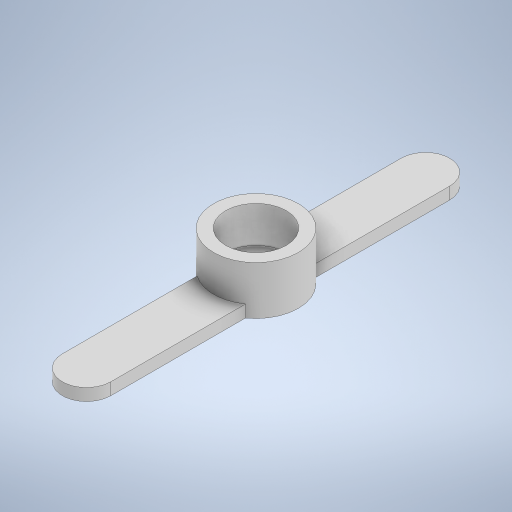
# Autodesk Inventor part: ServoWings
Saved by Autodesk Inventor 2024.2 (Build 282272000, 272)
## iProperties
Created: 2024-05-04
Part Number: ServoWings
Material: Generic
Document SubType Name: Modeling
Designer: ringl
Density: 1 g/cm^3
Appearance: Default
Author: ringl
Autodesk Inventor part; units mm, degrees
ref_plane "YZ Plane" through (0, 0, 0) normal (1, 0, 0) x (0, 1, 0)
ref_plane "XZ Plane" through (0, 0, 0) normal (0, 1, 0) x (-1, 0, 0)
ref_plane "XY Plane" through (0, 0, 0) normal (0, 0, 1) x (1, 0, 0)
sketch "Sketch1" plane through (0, 0, 0) normal (0, 1, 0) x (-1, 0, 0)
  line L0 (0, 0) -> (4, 0)
  line L1 (4, 0) -> (4, -32)
  line L2 (4, -32) -> (0, -32)
  line L3 (0, -32) -> (0, 0)
  dimension "d0" = 4
  dimension "d1" = 32
  constraints: 8 end point, 2 parallel, 1 horizontal, 1 perpendicular
  measures "d0" distance of L1.end L2.end
  measures "d1" distance of L0.end L1.end
extrude "Extrusion1" add sketch "Sketch1" along normal blind 1
fillet "Fillet1" radius 2 4 edges at (0, 0.5, 0) (-4, 0.5, 0) (0, 0.5, -32) (-4, 0.5, -32)
sketch "Sketch2" plane through (0, 1, 0) normal (0, 1, 0) x (1, 0, 0)
  circle A0 centre (-2, 16) radius 3.5
  arc A1 (-4, 2) -> (0, 2) centre (-2, 2) ccw projected
  line L0 (0, 2) -> (0, 30) projected
  point P0 (0, 0)
  point P1 (-2, 0)
  dimension "d5" = 7
  dimension "d6" = 16
  dimension "d7" = 2
  constraints: 1 centre point, 1 point on circle
  measures "d5" diameter of A0
  measures "d6" distance of point (-2, 0) A0.centre
  measures "d7" distance from line of L0 A0.centre
extrude "Extrusion2" add sketch "Sketch2" along normal blind 3
sketch "Sketch3" plane through (0, 1, 0) normal (0, -1, 0) x (1, 0, 0)
  line L0 (0, -13.1277) -> (0, -18.8723) projected
  arc A0 (0, -18.8723) -> (0, -13.1277) centre (-2, -16) ccw projected
  line L1 (-4, -18.8723) -> (-4, -13.1277) projected
  arc A1 (-4, -13.1277) -> (-4, -18.8723) centre (-2, -16) ccw projected
  arc A2 (0, -18.8723) -> (0, -13.1277) centre (-2, -16) ccw
  arc A3 (-4, -13.1277) -> (-4, -18.8723) centre (-2, -16) ccw
  line L2 (-4, -13.1277) -> (-4, -18.8723)
  line L3 (-4, -30) -> (-4, -2) projected
  line L4 (0, -13.1277) -> (0, -18.8723)
  line L5 (0, -2) -> (0, -30) projected
  point P0 (0, 0)
  constraints: 5 point on circle, 4 end point, 2 centre point, 2 collinear, 2 concentric, 1 point on line
extrude "Extrusion3" add sketch "Sketch3" along normal blind 1
sketch "Sketch4" plane through (0, 0, 0) normal (0, -1, 0) x (1, 0, 0)
  arc A0 (-4, -30) -> (0, -30) centre (-2, -30) ccw projected
  line L0 (0, -18.8723) -> (0, -30) projected
  arc A1 (0, -18.8723) -> (0, -13.1277) centre (-2, -16) ccw projected
  line L1 (0, -2) -> (0, -13.1277) projected
  arc A2 (0, -2) -> (-4, -2) centre (-2, -2) ccw projected
  line L2 (-4, -13.1277) -> (-4, -2) projected
  arc A3 (-4, -13.1277) -> (-4, -18.8723) centre (-2, -16) ccw projected
  line L3 (-4, -30) -> (-4, -18.8723) projected
  circle A4 centre (-2, -16) radius 1
  point P0 (0, 0)
  dimension "d12" = 2
  constraints: 1 centre point, 1 coincident
  measures "d12" diameter of A4
extrude "Extrusion4" cut sketch "Sketch4" against normal through all contours A4
sketch "Sketch5" plane through (-2, 4, -16) normal (0, 1, 0) x (1, 0, 0)
  circle A0 centre (0, 0) radius 1 projected
  circle A1 centre (0, 0) radius 2.5
  point P0 (2, -16)
  dimension "d15" = 5
  constraints: 1 centre point, 1 coincident
  measures "d15" diameter of A1
extrude "Extrusion5" cut sketch "Sketch5" against normal blind 3
body "Solid1"
